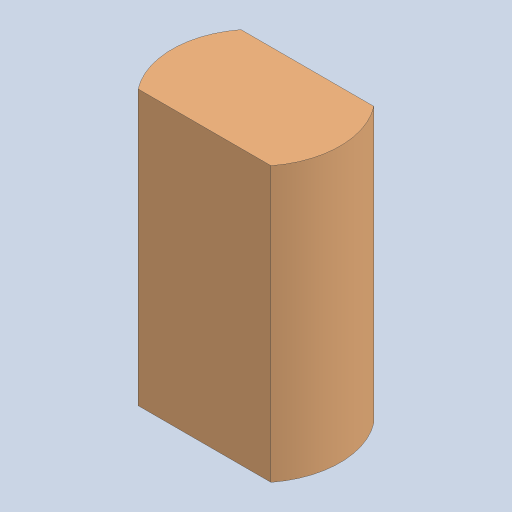
# Autodesk Inventor part: motor_axle
Saved by Autodesk Inventor 2024.4 (Build 284460000, 460)
## iProperties
Created: 2026-07-13
Part Number: motor_axle
Material: Generic
Document SubType Name: Modeling
Designer: tooles01
Density: 1 g/cm^3
Appearance: Default
Author: tooles01
Autodesk Inventor part; units mm, degrees
ref_plane "YZ Plane" through (0, 0, 0) normal (1, 0, 0) x (0, 1, 0)
ref_plane "XZ Plane" through (0, 0, 0) normal (0, 1, 0) x (-1, 0, 0)
ref_plane "XY Plane" through (0, 0, 0) normal (0, 0, 1) x (1, 0, 0)
sketch "Sketch1" plane through (0, 0, 0) normal (0, 1, 0) x (-1, 0, 0)
  circle A0 centre (0, 0) radius 2.45
  line L0 (1.9371, 1.5) -> (-1.9371, 1.5)
  line L1 (1.9371, -1.5) -> (-1.9371, -1.5)
  point P0 (0, -1.5)
  point P1 (0, 1.5)
  dimension "d0" = 3
  dimension "d1" = 4.9
  constraints: 4 end point, 4 point on circle, 2 midpoint, 2 vertical alignment, 1 centre point, 1 coincident, 1 horizontal, 1 parallel
  measures "d0" distance between parallel lines of L0 L1
  measures "d1" diameter of A0
extrude "Extrusion1" add sketch "Sketch1" along normal blind 8 contours A0 L1 L0
body "Solid1"
